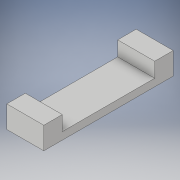
# Autodesk Inventor part: Loop
Saved by Autodesk Inventor 2019 (Build 230136000, 136)
## iProperties
Created: 2019-05-05
Part Number: Loop
Material: Generic
Document SubType Name: Modeling
Designer: Henry
Density: 1 g/cm^3
Appearance: Default
Author: Henry
Autodesk Inventor part; units mm, degrees
ref_plane "YZ Plane" through (0, 0, 0) normal (1, 0, 0) x (0, 1, 0)
ref_plane "XZ Plane" through (0, 0, 0) normal (0, 1, 0) x (-1, 0, 0)
ref_plane "XY Plane" through (0, 0, 0) normal (0, 0, 1) x (1, 0, 0)
sketch "Sketch1" plane through (0, 0, 0) normal (0, 1, 0) x (-1, 0, 0)
  line L0 (0, 0) -> (10.0076, 0)
  line L1 (10.0076, 0) -> (10.0076, -35.0012)
  line L2 (10.0076, -35.0012) -> (0, -35.0012)
  line L3 (0, -35.0012) -> (0, 0)
  dimension "d0" = 10.0076
  dimension "d1" = 35.0012
  constraints: 8 end point, 2 parallel, 1 horizontal, 1 perpendicular
  measures "d0" distance of L1.end L2.end
  measures "d1" distance of L0.end L1.end
extrude "Extrusion1" add sketch "Sketch1" along normal blind 2.0066
sketch "Sketch2" plane through (0, 2.0066, 0) normal (0, 1, 0) x (1, 0, 0)
  line L0 (-10.0076, 35.0012) -> (-10.0076, 0) projected
  line L1 (0, 0) -> (-10.0076, 0)
  line L2 (-10.0076, 0) -> (-10.0076, 5.0038)
  line L3 (-10.0076, 5.0038) -> (0, 5.0038)
  line L4 (0, 5.0038) -> (0, 0)
  line L5 (0, 0) -> (0, 35.0012) projected
  line L6 (0, 35.0012) -> (-10.0076, 35.0012)
  line L7 (-10.0076, 35.0012) -> (-10.0076, 29.9974)
  line L8 (-10.0076, 29.9974) -> (0, 29.9974)
  line L9 (0, 29.9974) -> (0, 35.0012)
  dimension "d4" = 5.0038
  dimension "d5" = 5.0038
  constraints: 16 end point, 4 parallel, 2 horizontal, 2 perpendicular, 2 point on line
  measures "d4" distance of L1.end L2.end
  measures "d5" distance of L7.end L6.end
extrude "Extrusion2" add sketch "Sketch2" along normal blind 3.9878 contours L6 L5 L8 L0 | L3 L4 L1 L0
body "Solid1"
